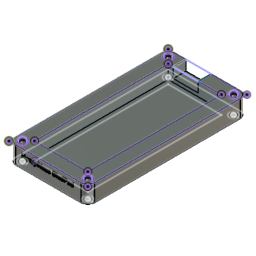
Hackpad Assembled (Autodesk Fusion 360 archive; units mm, degrees)
design "Hackpad case"
part number: 2026-03-30-20-08-03-036
Autodesk Fusion 360 part; units mm, degrees
sketch "CaseBase" plane through (0, 0, 0) normal (0, 0, 1) x (1, 0, 0)
  line L0 (0, 0) -> (39.45, 0)
  line L1 (39.45, 0) -> (39.45, 99)
  line L2 (39.45, 99) -> (0, 99)
  line L3 (0, 99) -> (0, 0)
  line L4 (48.95, 108.5) -> (-9.5, 108.5)
  line L5 (-9.5, 108.5) -> (-9.5, -9.5)
  line L6 (-9.5, -9.5) -> (48.95, -9.5)
  line L7 (48.95, -9.5) -> (48.95, 108.5)
  circle A0 centre (-4.5, 103.5) radius 1.7
  circle A1 centre (-4.5, -4.5) radius 1.7
  circle A2 centre (43.95, -4.5) radius 1.7
  circle A3 centre (43.95, 103.5) radius 1.7
  circle A4 centre (43.95, 103.5) radius 3
  circle A5 centre (-4.5, 103.5) radius 3
  circle A6 centre (43.95, -4.5) radius 3
  circle A7 centre (-4.5, -4.5) radius 3
  dimension "d1" = 99
  dimension "d2" = 39.45
  dimension "d3" = 58.45
  dimension "d4" = 118
  dimension "d5" = 9.5
  dimension "d6" = 9.5
  dimension "d7" = 3.4
  dimension "d8" = 3.4
  dimension "d9" = 3.4
  dimension "d10" = 3.4
  dimension "d11" = 5
  dimension "d12" = 5
  dimension "d13" = 5
  dimension "d14" = 5
  dimension "d15" = 5
  dimension "d16" = 5
  dimension "d17" = 5
  dimension "d18" = 5
  dimension "d19" = 6
  dimension "d20" = 6
  dimension "d21" = 6
  dimension "d22" = 6
  constraint horizontal L0
  constraint vertical L1
  constraint horizontal L2
  constraint vertical L3
  constraint coincident L0.start L3.end
  constraint horizontal L4
  constraint vertical L5
  constraint horizontal L6
  constraint vertical L7
  constraint concentric A3 A4
  constraint concentric A0 A5
  constraint concentric A2 A6
  constraint concentric A1 A7
  measures "d1" distance of L0.start L2.end
  measures "d2" distance of L1.end L2.end
  measures "d3" distance of L4.start L4.end
  measures "d4" distance of L4.start L6.end
  measures "d5" distance of L2 L4
  measures "d6" distance of L3 L5
  measures "d7" diameter of A0
  measures "d8" diameter of A1
  measures "d9" diameter of A2
  measures "d10" diameter of A3
  measures "d11" distance of L5 A0.centre
  measures "d12" distance of L4 A0.centre
  measures "d13" distance of L4 A3.centre
  measures "d14" distance of L7 A3.centre
  measures "d15" distance of L6 A2.centre
  measures "d16" distance of L7 A2.centre
  measures "d17" distance of L5 A1.centre
  measures "d18" distance of L6 A1.centre
  measures "d19" diameter of A4
  measures "d20" diameter of A5
  measures "d21" diameter of A6
  measures "d22" diameter of A7
extrude "Extrude1" add sketch "CaseBase" along normal blind 9.1 from surface at 3.1 contours A4 | A5 | A6 | A7 makes body 1 at (46.9351, -4.7987, 6.1333) makes body 2 at (-1.6809, 102.4739, 9.1667) makes body 3 at (-1.5149, -4.7987, 6.1333) makes body 4 at (41.1309, 102.4739, 9.1667)
extrude "Extrude2" add sketch "CaseBase" along normal blind 13 contours L4 L5 L6 L7 bodies 1 2 3 4
extrude "Extrude3" add sketch "CaseBase" along normal blind 3 contours L0 L1 L2 L3 bodies 1
sketch "USB" plane through (0, 0, 13) normal (0, 0, 1) x (1, 0, 0)
  line L0 (3.75, 108.5) -> (22.25, 108.5)
  line L1 (22.25, 108.5) -> (22.25, 99)
  line L2 (22.25, 99) -> (3.75, 99)
  line L3 (3.75, 99) -> (3.75, 108.5)
  line L4 (-9.5, 108.5) -> (-9.5, -9.5)
  circle A0 centre (43.95, 103.5) radius 3
  line L5 (0, 0) -> (0, 99)
  line L6 (0, 99) -> (39.45, 99)
  line L7 (39.45, 99) -> (39.45, 0)
  line L8 (39.45, 0) -> (0, 0)
  circle A1 centre (-4.5, -4.5) radius 3
  circle A2 centre (-4.5, 103.5) radius 3
  circle A3 centre (43.95, -4.5) radius 3
  line L9 (48.95, -9.5) -> (48.95, 108.5)
  line L10 (48.95, 108.5) -> (-9.5, 108.5)
  line L11 (-9.5, 108.5) -> (-9.5, -9.5)
  line L12 (-9.5, -9.5) -> (48.95, -9.5)
  dimension "d31" = 13.25
  constraint horizontal L0
  constraint vertical L1
  constraint horizontal L2
  constraint vertical L3
  measures "d31" distance of L3 L4
extrude "Extrude4" cut sketch "USB" against normal blind 7.5 contours L0 L1 L2 L3 L6 L10 bodies 1
fillet "Fillet1" radius 5 4 edges at (-9.5, 108.5, 6.5) (48.95, 108.5, 6.5) (-9.5, -9.5, 6.5) (48.95, -9.5, 6.5) on bodies 1
sketch "Branding" plane through (0, -9.5, 0) normal (0, -1, 0) x (1, 0, 0)
  line L0 (43.95, 0) -> (43.95, 13)
  line L1 (43.95, 13) -> (-4.5, 13)
  line L2 (-4.5, 13) -> (-4.5, 0)
  line L3 (-4.5, 0) -> (43.95, 0)
  line L4 (0, 5) -> (40, 5) construction
  line L5 (40, 5) -> (40, 10) construction
  line L6 (40, 10) -> (0, 10) construction
  line L7 (0, 10) -> (0, 5) construction
  dimension "d36" = 3
  text T0 "HenryWaus BludPad" font "Arial" height 3 align left top in box 40 x 5 at (0, 5) x (1, 0) y (0, 1) spacing 1 kerned
extrude "Extrude5" cut sketch "Branding" against normal blind 0.2 text T0 bodies 1
sketch "PCB" plane through (0, 0, 3) normal (0, 0, 1) x (-1, 0, 0)
  line L0 (0, -99) -> (0, 0)
  line L1 (0, 0) -> (-39.45, 0)
  line L2 (-39.45, 0) -> (-39.45, -99)
  line L3 (-39.45, -99) -> (0, -99)
  line L4 (0, -99) -> (-38.5, -99)
  line L5 (-38.5, -99) -> (-38.5, -1.2)
  line L6 (-38.5, -1.2) -> (0, -1.2)
  line L7 (0, -1.2) -> (0, -99)
  dimension "d40" = 97.8
  dimension "d41" = 38.5
  constraint horizontal L4
  constraint vertical L5
  constraint horizontal L6
  constraint vertical L7
  constraint coincident L0.start L3.end
  measures "d40" distance of L0.start L6.end
  measures "d41" distance of L5 L7
equation "d37 = 'HenryWaus BludPad'"
